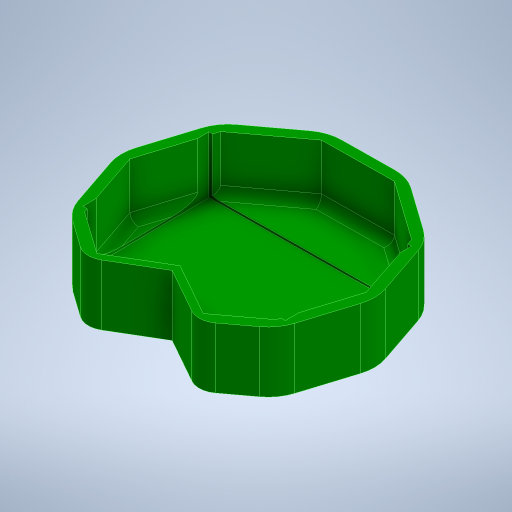
# Autodesk Inventor part: ShellMockup_01
Saved by Autodesk Inventor 2024 (Build 280153000, 153)
## iProperties
Created: 2023-11-09
Part Number: ShellMockup_01
Material: PLA
Document SubType Name: Modeling
Designer: jevan
Density: 1 g/cm^3
Appearance: Generic
Author: jevan
Autodesk Inventor part; units mm, degrees
ref_plane "YZ Plane" through (0, 0, 0) normal (1, 0, 0) x (0, 1, 0)
ref_plane "XZ Plane" through (0, 0, 0) normal (0, 1, 0) x (-1, 0, 0)
ref_plane "XY Plane" through (0, 0, 0) normal (0, 0, 1) x (1, 0, 0)
sketch "Sketch3" plane through (0, 0, 0) normal (0, 0, 1) x (1, 0, 0)
  line L0 (9.734, 29.9583) -> (25.484, 18.5152)
  line L1 (25.484, 18.5152) -> (31.5, 0)
  line L2 (31.5, 0) -> (25.484, -18.5152)
  line L3 (25.484, -18.5152) -> (9.734, -29.9583)
  line L4 (9.734, -29.9583) -> (-9.734, -29.9583)
  line L5 (-9.734, -29.9583) -> (-25.484, -18.5152)
  line L6 (-25.484, -18.5152) -> (-31.5, 0)
  line L7 (-31.5, 0) -> (-25.484, 18.5152)
  line L8 (-25.484, 18.5152) -> (-9.734, 29.9583)
  line L9 (-9.734, 29.9583) -> (9.734, 29.9583)
  line L10 (0, 29.9583) -> (0, 0)
  line L11 (-13.8564, 26.9632) -> (0, 18.9632)
  line L12 (0, 18.9632) -> (13.8564, 26.9632)
  line L13 (-8.9217, 27.4583) -> (-23.3574, 16.9702)
  line L14 (-23.3574, 16.9702) -> (-28.8713, 0)
  line L15 (-28.8713, 0) -> (-23.3574, -16.9702)
  line L16 (-23.3574, -16.9702) -> (-8.9217, -27.4583)
  line L17 (-8.9217, -27.4583) -> (8.9217, -27.4583)
  line L18 (8.9217, -27.4583) -> (23.3574, -16.9702)
  line L19 (23.3574, -16.9702) -> (28.8713, 0)
  line L20 (28.8713, 0) -> (23.3574, 16.9702)
  line L21 (23.3574, 16.9702) -> (8.9217, 27.4583)
  line L22 (8.9217, 27.4583) -> (-8.9217, 27.4583)
  line L23 (-13.3752, 24.7224) -> (0, 17.0002)
  line L24 (0, 17.0002) -> (13.3752, 24.7224)
  point P0 (12.9919, 24.5011)
  point P1 (-12.9919, 24.5011)
  dimension "d22" = 63
  dimension "d23" = 16
  dimension "d24" = 2.5
  dimension "d25" = 1.7
  dimension "d26" = 120
  constraints: 50 end point, 3 point on line, 1 coincident, 1 equal length, 1 midpoint, 1 vertical, 31 other
  measures "d22" distance of L1.end L6.end
  measures "d23" distance of L11.start L11.end
  measures "d24" distance between parallel lines of L8 L13
  measures "d25" distance between parallel lines of L11 L23
  measures "d26" angle of L12 L11
extrude "Extrusion3" add sketch "Sketch3" along normal blind 1.5 contours L0 L1 L2 L3 L4 L5 L6 L7 L8 L11 L13 L14 L15 L16 L17 L18 L19 L20 L21 L12 | L21 L24 L10 L12 | L10 L23 L13 L11 | L21 L20 L19 L18 L17 L16 L15 L14 L13 L23 L24
extrude "Extrusion4" add sketch "Sketch3" along normal blind 15 contours L0 L1 L2 L3 L4 L5 L6 L7 L8 L11 L13 L14 L15 L16 L17 L18 L19 L20 L21 L12 | L21 L24 L10 L12 | L10 L23 L13 L11
sketch "Sketch4" plane through (0, 0, 1.5) normal (0, 0, 1) x (1, 0, 0)
  line L0 (8.9217, -27.4583) -> (-8.9217, -27.4583) projected
  line L1 (0, -27.4583) -> (0, -14.7583)
  line L2 (-24, 15.2417) -> (24, 15.2417)
  line L3 (24, 15.2417) -> (24, -14.7583)
  line L4 (24, -14.7583) -> (-24, -14.7583)
  line L5 (-24, -14.7583) -> (-24, 15.2417)
  line L6 (24.75, 15.9917) -> (-24.75, 15.9917)
  line L7 (-24.75, 15.9917) -> (-24.75, -15.5083)
  line L8 (-24.75, -15.5083) -> (24.75, -15.5083)
  line L9 (24.75, -15.5083) -> (24.75, 15.9917)
  point P0 (0, 0)
  dimension "d31" = 12.7
  dimension "d32" = 48
  dimension "d33" = 30
  dimension "d36" = 0.75
  constraints: 18 end point, 4 parallel, 2 midpoint, 2 perpendicular, 1 horizontal, 1 vertical, 3 other
  measures "d31" distance of L1.end L1.start
  measures "d32" distance of L3.end L4.end
  measures "d33" distance of L4.end L2.start
  measures "d36" distance between parallel lines of L2 L6
extrude "Extrusion5" cut sketch "Sketch4" along normal blind 13.5 and the other way blind 0.6 contours L2 L3 L4 L5 | L9 L8 L7 L6
fillet "Fillet1" radius 10 8 edges at (-25.484, 18.5152, 7.5) (-31.5, 0, 7.5) (-25.484, -18.5152, 7.5) (-9.734, -29.9583, 7.5) (9.734, -29.9583, 7.5) (25.484, -18.5152, 7.5) (31.5, 0, 7.5) (25.484, 18.5152, 7.5)
fillet "Fillet2" radius 2 11 edges at (-18.1747, 20.7356, 1.5) (-26.8107, 6.3421, 1.5) (-26.8107, -6.3421, 1.5) (-16.1396, -22.2142, 1.5) (0, -27.4583, 1.5) (16.1396, -22.2142, 1.5) (26.8107, -6.3421, 1.5) (26.8107, 6.3421, 1.5) (18.1747, 20.7356, 1.5) (6.496, 20.7507, 1.5) (-6.496, 20.7507, 1.5)
fillet "Fillet5" radius 5 2 edges at (-13.8564, 26.9632, 7.5) (13.8564, 26.9632, 7.5)
body "Solid2"
